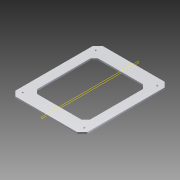
# Autodesk Inventor part: D-053
Saved by Autodesk Inventor 2015 (Build 190159000, 159)
## iProperties
Company: MARCHA TECHNOLOGY
Created: 2013-10-01
Part Number: D-053
Document SubType Name: Modeling
Designer: O.Martin
Density: 1.06 g/cm^3
Material: ABS Plastic
Mass: 612.404 g
Surface Area: 1658.31 cm^2
Volume: 577.739 cm^3
Project: WITBOXprinter_K01
Description: LATERAL IZQUIERDO
Stock Number: 28656
Appearance: Cool White
Author: O.Martin
Autodesk Inventor part; units mm, degrees
ref_plane "XZ Plane" through (0, 0, 0) normal (0, 1, 0) x (-1, 0, 0)
ref_plane "XY Plane" through (0, 0, 0) normal (0, 0, 1) x (1, 0, 0)
sketch "Boceto1" plane through (0, 0, 0) normal (0, 0, 1) x (1, 0, 0)
  line L0 (-179.5, 218.25) -> (179.5, 218.25)
  line L1 (179.5, 218.25) -> (179.5, -218.25)
  line L2 (179.5, -218.25) -> (-179.5, -218.25)
  line L3 (-179.5, -218.25) -> (-179.5, 218.25)
  line L4 (-112, 153.25) -> (112, 153.25)
  line L5 (132, 133.25) -> (132, -133.25)
  line L6 (112, -153.25) -> (-112, -153.25)
  line L7 (-132, -133.25) -> (-132, 133.25)
  line L8 (112, 153.25) -> (132, 133.25)
  line L9 (-132, -133.25) -> (-112, -153.25)
  line L10 (-132, 133.25) -> (-112, 153.25)
  line L11 (-179.5, 193.25) -> (-154.5, 218.25)
  line L12 (179.5, 193.25) -> (154.5, 218.25)
  line L13 (-179.5, -193.25) -> (-154.5, -218.25)
  line L14 (179.5, -193.25) -> (154.5, -218.25)
  line L15 (132, -133.25) -> (112, -153.25)
  point P0 (0, 0)
  point P1 (0, 218.25)
  point P2 (179.5, 0)
  point P3 (0, 153.25)
  dimension "d0" = 359
  dimension "d1" = 436.5
  dimension "d4" = 65
  dimension "d7" = 45
  dimension "d8" = 20
  dimension "d9" = 25
  dimension "d15" = 47.5
  dimension "d20" = 65
  constraints: 32 end point, 8 parallel, 8 point on line, 6 equal length, 5 perpendicular, 3 midpoint, 2 horizontal, 2 vertical alignment, 1 horizontal alignment
  measures "d0" distance of L0.start L0.end
  measures "d1" distance of L0.end L1.end
  measures "d4" distance between parallel lines of L2 L6
  measures "d7" angle of L5 L8
  measures "d8" horizontal distance of L7.end L4.start
  measures "d9" horizontal distance of L11.start L11.end
  measures "d15" distance between parallel lines of L3 L7
  measures "d20" distance between parallel lines of L0 L4
extrude "Extrusión1" add sketch "Boceto1" along normal blind 8 contours L0 L12 L1 L14 L2 L13 L3 L11
fillet "Empalme1" radius 10 8 edges at (-112, 153.25, 4) (112, 153.25, 4) (132, 133.25, 4) (-132, 133.25, 4) (132, -133.25, 4) (112, -153.25, 4) (-112, -153.25, 4) (-132, -133.25, 4)
chamfer "Chaflán1" [suppressed]
sketch "Boceto3" plane through (0, 0, 8) normal (0, 0, 1) x (1, 0, 0)
  line L0 (-153.5, 182.25) -> (153.5, 182.25) construction
  line L1 (153.5, 182.25) -> (153.5, -182.25) construction
  line L2 (153.5, -182.25) -> (-153.5, -182.25) construction
  line L3 (-153.5, -182.25) -> (-153.5, 182.25) construction
  line L4 (-129.0711, 136.1789) -> (-114.9289, 150.3211) projected
  arc A0 (-107.8579, 153.25) -> (-114.9289, 150.3211) centre (-107.8579, 143.25) ccw projected
  line L5 (-107.8579, 153.25) -> (107.8579, 153.25) projected
  arc A1 (114.9289, 150.3211) -> (107.8579, 153.25) centre (107.8579, 143.25) ccw projected
  line L6 (114.9289, 150.3211) -> (129.0711, 136.1789) projected
  arc A2 (132, 129.1079) -> (129.0711, 136.1789) centre (122, 129.1079) ccw projected
  line L7 (132, 129.1079) -> (132, -129.1079) projected
  arc A3 (129.0711, -136.1789) -> (132, -129.1079) centre (122, -129.1079) ccw projected
  line L8 (129.0711, -136.1789) -> (114.9289, -150.3211) projected
  arc A4 (107.8579, -153.25) -> (114.9289, -150.3211) centre (107.8579, -143.25) ccw projected
  line L9 (107.8579, -153.25) -> (-107.8579, -153.25) projected
  arc A5 (-114.9289, -150.3211) -> (-107.8579, -153.25) centre (-107.8579, -143.25) ccw projected
  line L10 (-114.9289, -150.3211) -> (-129.0711, -136.1789) projected
  arc A6 (-132, -129.1079) -> (-129.0711, -136.1789) centre (-122, -129.1079) ccw projected
  line L11 (-132, -129.1079) -> (-132, 129.1079) projected
  arc A7 (-129.0711, 136.1789) -> (-132, 129.1079) centre (-122, 129.1079) ccw projected
  line L12 (-179.5, 193.25) -> (-154.5, 218.25) projected
  line L13 (-179.5, -193.25) -> (-179.5, 193.25) projected
  line L14 (-154.5, -218.25) -> (-179.5, -193.25) projected
  line L15 (154.5, -218.25) -> (-154.5, -218.25) projected
  line L16 (179.5, -193.25) -> (154.5, -218.25) projected
  line L17 (179.5, 193.25) -> (179.5, -193.25) projected
  line L18 (154.5, 218.25) -> (179.5, 193.25) projected
  line L19 (-154.5, 218.25) -> (154.5, 218.25) projected
  line L20 (179.5, 193.25) -> (179.5, -193.25) projected
  line L21 (-154.5, 218.25) -> (154.5, 218.25) projected
  point P0 (0, 182.25)
  point P1 (153.5, 0)
  point P2 (179.5, 0)
  point P3 (0, 218.25)
  dimension "d36" = 307
  dimension "d37" = 364.5
  constraints: 8 end point, 4 coincident, 4 midpoint, 2 parallel, 1 horizontal, 1 horizontal alignment, 1 perpendicular, 1 vertical alignment
  measures "d36" distance of L0.start L0.end
  measures "d37" distance of L0.end L1.end
hole "Agujero1" at (-153.5, 182.25, 8) at (153.5, 182.25, 8) at (153.5, -182.25, 8) at (-153.5, -182.25, 8) direction (0, 0, -1) diameter 7 end through all
sketch "Boceto5" plane through (0, 0, 0) normal (0, 0, -1) x (-1, 0, 0)
  line L0 (154.5, 218.25) -> (179.5, 193.25) projected
  line L1 (-154.5, 218.25) -> (154.5, 218.25) projected
  line L2 (-179.5, 193.25) -> (-154.5, 218.25) projected
  line L3 (154.5, -218.25) -> (-154.5, -218.25) projected
  line L4 (-162.5, 210.25) -> (162.5, 210.25)
  dimension "d33" = 8
  constraints: 2 end point, 2 point on line, 1 parallel
  measures "d33" distance between parallel lines of L1 L4
sketch "Boceto4" plane through (0, 0, 0) normal (0, 0, -1) x (-1, 0, 0)
  line L0 (114.9289, 150.3211) -> (129.0711, 136.1789) projected
  arc A0 (132, 129.1079) -> (129.0711, 136.1789) centre (122, 129.1079) ccw projected
  line L1 (132, 129.1079) -> (132, -129.1079) projected
  arc A1 (129.0711, -136.1789) -> (132, -129.1079) centre (122, -129.1079) ccw projected
  line L2 (129.0711, -136.1789) -> (114.9289, -150.3211) projected
  arc A2 (107.8579, -153.25) -> (114.9289, -150.3211) centre (107.8579, -143.25) ccw projected
  line L3 (107.8579, -153.25) -> (-107.8579, -153.25) projected
  arc A3 (-114.9289, -150.3211) -> (-107.8579, -153.25) centre (-107.8579, -143.25) ccw projected
  line L4 (-114.9289, -150.3211) -> (-129.0711, -136.1789) projected
  arc A4 (-132, -129.1079) -> (-129.0711, -136.1789) centre (-122, -129.1079) ccw projected
  line L5 (-132, -129.1079) -> (-132, 129.1079) projected
  arc A5 (-129.0711, 136.1789) -> (-132, 129.1079) centre (-122, 129.1079) ccw projected
  line L6 (-129.0711, 136.1789) -> (-114.9289, 150.3211) projected
  arc A6 (-107.8579, 153.25) -> (-114.9289, 150.3211) centre (-107.8579, 143.25) ccw projected
  line L7 (-107.8579, 153.25) -> (107.8579, 153.25) projected
  arc A7 (114.9289, 150.3211) -> (107.8579, 153.25) centre (107.8579, 143.25) ccw projected
  line L8 (107.8579, 163.25) -> (-107.8579, 163.25)
  arc A8 (-107.8579, 163.25) -> (-122, 157.3921) centre (-107.8579, 143.25) ccw
  line L9 (-122, 157.3921) -> (-136.1421, 143.25)
  arc A9 (-136.1421, 143.25) -> (-142, 129.1079) centre (-122, 129.1079) ccw
  line L10 (-142, 129.1079) -> (-142, -129.1079)
  arc A10 (-142, -129.1079) -> (-136.1421, -143.25) centre (-122, -129.1079) ccw
  line L11 (-136.1421, -143.25) -> (-122, -157.3921)
  arc A11 (-122, -157.3921) -> (-107.8579, -163.25) centre (-107.8579, -143.25) ccw
  line L12 (-107.8579, -163.25) -> (107.8579, -163.25)
  arc A12 (107.8579, -163.25) -> (122, -157.3921) centre (107.8579, -143.25) ccw
  line L13 (122, -157.3921) -> (136.1421, -143.25)
  arc A13 (136.1421, -143.25) -> (142, -129.1079) centre (122, -129.1079) ccw
  line L14 (142, -129.1079) -> (142, 129.1079)
  arc A14 (142, 129.1079) -> (136.1421, 143.25) centre (122, 129.1079) ccw
  line L15 (136.1421, 143.25) -> (122, 157.3921)
  arc A15 (122, 157.3921) -> (107.8579, 163.25) centre (107.8579, 143.25) ccw
  dimension "d30" = 10
  constraints: 16 end point, 16 point on circle, 8 centre point, 15 other
  measures "d30" distance between parallel lines of L7 L8
body "Solid1"
